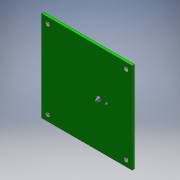
# Autodesk Inventor part: Patch_Antenna_V1
Saved by Autodesk Inventor 2016 (Build 200138000, 138)
## iProperties
Created: 2016-11-19
Part Number: Patch_Antenna_V1
Material: Generic
Document SubType Name: Modeling
Designer: Christopher
Density: 2.8165 g/cm^3
Appearance: Default
Mass: 13.509 g
Surface Area: 46.4955 cm^2
Volume: 4.79638 cm^3
Author: Christopher
Autodesk Inventor part; units mm, degrees
ref_plane "YZ Plane" through (0, 0, 0) normal (1, 0, 0) x (0, 1, 0)
ref_plane "XZ Plane" through (0, 0, 0) normal (0, 1, 0) x (-1, 0, 0)
sketch "Sketch1" plane through (0, 0, 0) normal (0, 1, 0) x (-1, 0, 0)
  line L0 (0, 0) -> (45, 0)
  line L1 (45, 0) -> (45, -45)
  line L2 (45, -45) -> (0, -45)
  line L3 (0, -45) -> (0, 0)
  dimension "d0" = 45
  dimension "d1" = 45
  constraints: 8 end point, 2 parallel, 1 horizontal, 1 perpendicular
  measures "d0" distance of L1.end L2.end
  measures "d1" distance of L0.end L1.end
extrude "Extrusion1" add sketch "Sketch1" along normal blind 1.15
sketch "Sketch2" plane through (0, 1.15, 0) normal (0, 1, 0) x (1, 0, 0)
  line L0 (-45, 45) -> (-45, 0) projected
  line L1 (-45, 0) -> (-45, 3)
  line L2 (-45, 3) -> (-42, 3)
  line L3 (-45, 22.5) -> (-42, 22.5)
  line L4 (-45, 45) -> (-45, 42)
  line L5 (-45, 42) -> (-42, 42)
  line L6 (0, 45) -> (-45, 45) projected
  line L7 (-22.5, 45) -> (-22.5, 42.897)
  line L8 (0, 45) -> (0, 0)
  line L9 (0, 0) -> (0, 3)
  line L10 (0, 3) -> (-3, 3)
  line L11 (0, 22.5) -> (-3, 22.5)
  line L12 (0, 45) -> (0, 42)
  line L13 (0, 42) -> (-3, 42)
  dimension "d4" = 3
  dimension "d5" = 3
  constraints: 24 end point, 9 symmetric about line, 2 midpoint, 2 point on line, 1 horizontal, 1 perpendicular, 1 vertical
  measures "d4" distance of L0.end L1.end
  measures "d5" distance of L1.end L2.end
hole "Hole1" at (-42, 1.15, -3) at (-42, 1.15, -42) at (-3, 1.15, -42) at (-3, 1.15, -3) direction (0, -1, 0) diameter 2.2 end through all clearance for "Flat Head Machine Screw" size "M2" standard "Ansi Metric M Profile"
sketch "Sketch3" plane through (0, 1.15, 0) normal (0, 1, 0) x (1, 0, 0)
  line L0 (-45, 0) -> (-45, 45) projected
  line L1 (0, 45) -> (0, 0) projected
  line L2 (-45, 45) -> (0, 45) projected
  line L3 (-35, 10) -> (-10, 10)
  line L4 (-10, 10) -> (-10, 35)
  line L5 (-10, 35) -> (-35, 35)
  line L6 (-35, 10) -> (-35, 35)
  dimension "d15" = 25
  dimension "d16" = 25
  dimension "d17" = 10
  dimension "d18" = 10
  dimension "d19" = 10
  constraints: 8 end point, 1 vertical
  measures "d15" distance of L3.start L3.end
  measures "d16" distance of L3.end L4.end
  measures "d17" distance between parallel lines of L2 L5
  measures "d18" distance between parallel lines of L0 L6
  measures "d19" distance between parallel lines of L1 L4
extrude "Extrusion2" add sketch "Sketch3" along normal blind 4
chamfer "Chamfer1" distance 1.5 angle 45 4 edges at (-10, 3.15, -35) (-35, 3.15, -35) (-10, 3.15, -10) (-35, 3.15, -10)
sketch "Sketch4" plane through (0, 0, 0) normal (0, -1, 0) x (1, 0, 0)
  line L0 (0, 0) -> (0, -45) projected
  line L1 (0, -22.5) -> (-12.5, -22.5)
  line L2 (-12.5, -22.5) -> (-16.5, -22.5)
  circle A0 centre (-12.5, -22.5) radius 0.5
  circle A1 centre (-16.5, -22.5) radius 0.5
  dimension "d25" = 12.5
  dimension "d26" = 4
  dimension "d27" = 1
  constraints: 4 end point, 2 centre point, 2 coincident, 2 horizontal, 1 midpoint
  measures "d25" distance of L1.start L1.end
  measures "d26" distance of L1.end L2.end
  measures "d27" diameter of A0
ref_plane "Work Plane1" through (-12.5, 0, -22.5) normal (0, 0, 1) x (-1, 0, 0)
sketch "Sketch5" plane through (-12.5, 0, -22.5) normal (0, 0, 1) x (-1, 0, 0)
  line L0 (0, 0) -> (4, 0) projected
  line L1 (-12.5, 0) -> (0, 0) projected
  line L2 (4, 0) -> (4, 2)
  line L3 (4, 0) -> (5.15, 0)
  line L4 (4, 2) -> (5.15, 0)
  line L5 (0, 0) -> (0.575, 0)
  point P0 (-12.5, 0)
  dimension "d31" = 2
  dimension "d33" = 1.15
  constraints: 8 end point, 1 horizontal, 1 point on line, 1 vertical
  measures "d31" distance of L0.end L2.end
  measures "d33" distance of L0.end L3.end
revolve "Revolution1" add sketch "Sketch5" angle 360 about axis through (-16.5, 0, -22.5) along (0, -1, 0)
sketch "Sketch6" plane through (-12.5, 0, -22.5) normal (0, 0, 1) x (-1, 0, 0)
  line L0 (0, 0) -> (0, 1)
  line L1 (0, 0) -> (0.575, 0)
  line L2 (0, 1) -> (0.575, 0)
  point P0 (-12.5, 0)
  dimension "d36" = 1
  dimension "d37" = 0.575
  constraints: 6 end point, 1 horizontal, 1 vertical
  measures "d36" distance of L0.start L0.end
  measures "d37" distance of L0.start L1.end
revolve "Revolution2" add sketch "Sketch6" angle 360 about axis through (-12.5, 0, -22.5) along (0, -1, 0)
body "Solid1"
